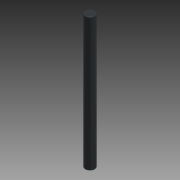
# Autodesk Inventor part: 1221_Center Former Shaft_V1
Saved by Autodesk Inventor 2020 (Build 240168000, 168)
## iProperties
Created: 2019-09-13
Part Number: 1221_Center Former Shaft_V1
Material: Iron, Gray
Document SubType Name: Modeling
Designer: MPI
Density: 7.15 g/cm^3
Appearance: Iron Gray
Mass: 172.281 g
Surface Area: 281.442 cm^2
Volume: 172.281 cm^3
Author: MPI
Autodesk Inventor part; units mm, degrees
ref_plane "YZ Plane" through (0, 0, 0) normal (1, 0, 0) x (0, 1, 0)
ref_plane "XZ Plane" through (0, 0, 0) normal (0, 1, 0) x (-1, 0, 0)
ref_plane "XY Plane" through (0, 0, 0) normal (0, 0, 1) x (1, 0, 0)
sketch "Sketch1" plane through (0, 0, 0) normal (0, 0, 1) x (1, 0, 0)
  circle A0 centre (0, 0) radius 12.7
  dimension "d0" = 25.4
  constraints: 1 centre point, 1 coincident
  measures "d0" diameter of A0
extrude "Extrusion1" add sketch "Sketch1" along normal blind 360
chamfer "Chamfer1" distance 1 angle 45 2 edges at (-12.7, 0, 360) (-12.7, 0, 0)
body "Solid1"
